Autodesk Fusion 360 part; units mm, degrees
(part 6 of 6)
  line L698 (-62.5, 150.325) -> (-62.5, 137.675)
  arc A698 (-65.675, 134.5) -> (-62.5, 137.675) centre (-65.675, 137.675) ccw
  line L699 (-65.675, 134.5) -> (-78.325, 134.5)
  arc A699 (-81.5, 137.675) -> (-78.325, 134.5) centre (-78.325, 137.675) ccw
  line L700 (-177.5, 137.675) -> (-177.5, 150.325)
  arc A700 (-174.325, 153.5) -> (-177.5, 150.325) centre (-174.325, 150.325) ccw
  line L701 (-174.325, 153.5) -> (-161.675, 153.5)
  arc A701 (-158.5, 150.325) -> (-161.675, 153.5) centre (-161.675, 150.325) ccw
  line L702 (-158.5, 150.325) -> (-158.5, 137.675)
  arc A702 (-161.675, 134.5) -> (-158.5, 137.675) centre (-161.675, 137.675) ccw
  line L703 (-161.675, 134.5) -> (-174.325, 134.5)
  arc A703 (-177.5, 137.675) -> (-174.325, 134.5) centre (-174.325, 137.675) ccw
  line L704 (-105.5, 113.675) -> (-105.5, 126.325)
  arc A704 (-102.325, 129.5) -> (-105.5, 126.325) centre (-102.325, 126.325) ccw
  line L705 (-102.325, 129.5) -> (-89.675, 129.5)
  arc A705 (-86.5, 126.325) -> (-89.675, 129.5) centre (-89.675, 126.325) ccw
  line L706 (-86.5, 126.325) -> (-86.5, 113.675)
  arc A706 (-89.675, 110.5) -> (-86.5, 113.675) centre (-89.675, 113.675) ccw
  line L707 (-89.675, 110.5) -> (-102.325, 110.5)
  arc A707 (-105.5, 113.675) -> (-102.325, 110.5) centre (-102.325, 113.675) ccw
  line L708 (-33.5, 89.675) -> (-33.5, 102.325)
  arc A708 (-30.325, 105.5) -> (-33.5, 102.325) centre (-30.325, 102.325) ccw
  line L709 (-30.325, 105.5) -> (-17.675, 105.5)
  arc A709 (-14.5, 102.325) -> (-17.675, 105.5) centre (-17.675, 102.325) ccw
  line L710 (-14.5, 102.325) -> (-14.5, 89.675)
  arc A710 (-17.675, 86.5) -> (-14.5, 89.675) centre (-17.675, 89.675) ccw
  line L711 (-17.675, 86.5) -> (-30.325, 86.5)
  arc A711 (-33.5, 89.675) -> (-30.325, 86.5) centre (-30.325, 89.675) ccw
  line L712 (-129.5, 89.675) -> (-129.5, 102.325)
  arc A712 (-126.325, 105.5) -> (-129.5, 102.325) centre (-126.325, 102.325) ccw
  line L713 (-126.325, 105.5) -> (-113.675, 105.5)
  arc A713 (-110.5, 102.325) -> (-113.675, 105.5) centre (-113.675, 102.325) ccw
  line L714 (-110.5, 102.325) -> (-110.5, 89.675)
  arc A714 (-113.675, 86.5) -> (-110.5, 89.675) centre (-113.675, 89.675) ccw
  line L715 (-113.675, 86.5) -> (-126.325, 86.5)
  arc A715 (-129.5, 89.675) -> (-126.325, 86.5) centre (-126.325, 89.675) ccw
  line L716 (-57.5, 65.675) -> (-57.5, 78.325)
  arc A716 (-54.325, 81.5) -> (-57.5, 78.325) centre (-54.325, 78.325) ccw
  line L717 (-54.325, 81.5) -> (-41.675, 81.5)
  arc A717 (-38.5, 78.325) -> (-41.675, 81.5) centre (-41.675, 78.325) ccw
  line L718 (-38.5, 78.325) -> (-38.5, 65.675)
  arc A718 (-41.675, 62.5) -> (-38.5, 65.675) centre (-41.675, 65.675) ccw
  line L719 (-41.675, 62.5) -> (-54.325, 62.5)
  arc A719 (-57.5, 65.675) -> (-54.325, 62.5) centre (-54.325, 65.675) ccw
  line L720 (-153.5, 65.675) -> (-153.5, 78.325)
  arc A720 (-150.325, 81.5) -> (-153.5, 78.325) centre (-150.325, 78.325) ccw
  line L721 (-150.325, 81.5) -> (-137.675, 81.5)
  arc A721 (-134.5, 78.325) -> (-137.675, 81.5) centre (-137.675, 78.325) ccw
  line L722 (-134.5, 78.325) -> (-134.5, 65.675)
  arc A722 (-137.675, 62.5) -> (-134.5, 65.675) centre (-137.675, 65.675) ccw
  line L723 (-137.675, 62.5) -> (-150.325, 62.5)
  arc A723 (-153.5, 65.675) -> (-150.325, 62.5) centre (-150.325, 65.675) ccw
  line L724 (-177.5, -54.325) -> (-177.5, -41.675)
  arc A724 (-174.325, -38.5) -> (-177.5, -41.675) centre (-174.325, -41.675) ccw
  line L725 (-174.325, -38.5) -> (-161.675, -38.5)
  arc A725 (-158.5, -41.675) -> (-161.675, -38.5) centre (-161.675, -41.675) ccw
  line L726 (-158.5, -41.675) -> (-158.5, -54.325)
  arc A726 (-161.675, -57.5) -> (-158.5, -54.325) centre (-161.675, -54.325) ccw
  line L727 (-161.675, -57.5) -> (-174.325, -57.5)
  arc A727 (-177.5, -54.325) -> (-174.325, -57.5) centre (-174.325, -54.325) ccw
  line L728 (-129.5, -102.325) -> (-129.5, -89.675)
  arc A728 (-126.325, -86.5) -> (-129.5, -89.675) centre (-126.325, -89.675) ccw
  line L729 (-126.325, -86.5) -> (-113.675, -86.5)
  arc A729 (-110.5, -89.675) -> (-113.675, -86.5) centre (-113.675, -89.675) ccw
  line L730 (-110.5, -89.675) -> (-110.5, -102.325)
  arc A730 (-113.675, -105.5) -> (-110.5, -102.325) centre (-113.675, -102.325) ccw
  line L731 (-113.675, -105.5) -> (-126.325, -105.5)
  arc A731 (-129.5, -102.325) -> (-126.325, -105.5) centre (-126.325, -102.325) ccw
  line L732 (-153.5, -126.325) -> (-153.5, -113.675)
  arc A732 (-150.325, -110.5) -> (-153.5, -113.675) centre (-150.325, -113.675) ccw
  line L733 (-150.325, -110.5) -> (-137.675, -110.5)
  arc A733 (-134.5, -113.675) -> (-137.675, -110.5) centre (-137.675, -113.675) ccw
  line L734 (-134.5, -113.675) -> (-134.5, -126.325)
  arc A734 (-137.675, -129.5) -> (-134.5, -126.325) centre (-137.675, -126.325) ccw
  line L735 (-137.675, -129.5) -> (-150.325, -129.5)
  arc A735 (-153.5, -126.325) -> (-150.325, -129.5) centre (-150.325, -126.325) ccw
  line L736 (-177.5, -150.325) -> (-177.5, -137.675)
  arc A736 (-174.325, -134.5) -> (-177.5, -137.675) centre (-174.325, -137.675) ccw
  line L737 (-174.325, -134.5) -> (-161.675, -134.5)
  arc A737 (-158.5, -137.675) -> (-161.675, -134.5) centre (-161.675, -137.675) ccw
  line L738 (-158.5, -137.675) -> (-158.5, -150.325)
  arc A738 (-161.675, -153.5) -> (-158.5, -150.325) centre (-161.675, -150.325) ccw
  line L739 (-161.675, -153.5) -> (-174.325, -153.5)
  arc A739 (-177.5, -150.325) -> (-174.325, -153.5) centre (-174.325, -150.325) ccw
  line L740 (38.5, -150.325) -> (38.5, -137.675)
  arc A740 (41.675, -134.5) -> (38.5, -137.675) centre (41.675, -137.675) ccw
  line L741 (41.675, -134.5) -> (54.325, -134.5)
  arc A741 (57.5, -137.675) -> (54.325, -134.5) centre (54.325, -137.675) ccw
  line L742 (57.5, -137.675) -> (57.5, -150.325)
  arc A742 (54.325, -153.5) -> (57.5, -150.325) centre (54.325, -150.325) ccw
  line L743 (54.325, -153.5) -> (41.675, -153.5)
  arc A743 (38.5, -150.325) -> (41.675, -153.5) centre (41.675, -150.325) ccw
  line L744 (-81.5, 41.675) -> (-81.5, 54.325)
  arc A744 (-78.325, 57.5) -> (-81.5, 54.325) centre (-78.325, 54.325) ccw
  line L745 (-78.325, 57.5) -> (-65.675, 57.5)
  arc A745 (-62.5, 54.325) -> (-65.675, 57.5) centre (-65.675, 54.325) ccw
  line L746 (-62.5, 54.325) -> (-62.5, 41.675)
  arc A746 (-65.675, 38.5) -> (-62.5, 41.675) centre (-65.675, 41.675) ccw
  line L747 (-65.675, 38.5) -> (-78.325, 38.5)
  arc A747 (-81.5, 41.675) -> (-78.325, 38.5) centre (-78.325, 41.675) ccw
  line L748 (38.5, -174.325) -> (38.5, -161.675)
  arc A748 (41.675, -158.5) -> (38.5, -161.675) centre (41.675, -161.675) ccw
  line L749 (41.675, -158.5) -> (54.325, -158.5)
  arc A749 (57.5, -161.675) -> (54.325, -158.5) centre (54.325, -161.675) ccw
  line L750 (57.5, -161.675) -> (57.5, -174.325)
  arc A750 (54.325, -177.5) -> (57.5, -174.325) centre (54.325, -174.325) ccw
  line L751 (54.325, -177.5) -> (41.675, -177.5)
  arc A751 (38.5, -174.325) -> (41.675, -177.5) centre (41.675, -174.325) ccw
  line L752 (-105.5, -150.325) -> (-105.5, -137.675)
  arc A752 (-102.325, -134.5) -> (-105.5, -137.675) centre (-102.325, -137.675) ccw
  line L753 (-102.325, -134.5) -> (-89.675, -134.5)
  arc A753 (-86.5, -137.675) -> (-89.675, -134.5) centre (-89.675, -137.675) ccw
  line L754 (-86.5, -137.675) -> (-86.5, -150.325)
  arc A754 (-89.675, -153.5) -> (-86.5, -150.325) centre (-89.675, -150.325) ccw
  line L755 (-89.675, -153.5) -> (-102.325, -153.5)
  arc A755 (-105.5, -150.325) -> (-102.325, -153.5) centre (-102.325, -150.325) ccw
  line L756 (-57.5, 41.675) -> (-57.5, 54.325)
  arc A756 (-54.325, 57.5) -> (-57.5, 54.325) centre (-54.325, 54.325) ccw
  line L757 (-54.325, 57.5) -> (-41.675, 57.5)
  arc A757 (-38.5, 54.325) -> (-41.675, 57.5) centre (-41.675, 54.325) ccw
  line L758 (-38.5, 54.325) -> (-38.5, 41.675)
  arc A758 (-41.675, 38.5) -> (-38.5, 41.675) centre (-41.675, 41.675) ccw
  line L759 (-41.675, 38.5) -> (-54.325, 38.5)
  arc A759 (-57.5, 41.675) -> (-54.325, 38.5) centre (-54.325, 41.675) ccw
  line L760 (-129.5, -30.325) -> (-129.5, -17.675)
  arc A760 (-126.325, -14.5) -> (-129.5, -17.675) centre (-126.325, -17.675) ccw
  line L761 (-126.325, -14.5) -> (-113.675, -14.5)
  arc A761 (-110.5, -17.675) -> (-113.675, -14.5) centre (-113.675, -17.675) ccw
  line L762 (-110.5, -17.675) -> (-110.5, -30.325)
  arc A762 (-113.675, -33.5) -> (-110.5, -30.325) centre (-113.675, -30.325) ccw
  line L763 (-113.675, -33.5) -> (-126.325, -33.5)
  arc A763 (-129.5, -30.325) -> (-126.325, -33.5) centre (-126.325, -30.325) ccw
  line L764 (-105.5, -102.325) -> (-105.5, -89.675)
  arc A764 (-102.325, -86.5) -> (-105.5, -89.675) centre (-102.325, -89.675) ccw
  line L765 (-102.325, -86.5) -> (-89.675, -86.5)
  arc A765 (-86.5, -89.675) -> (-89.675, -86.5) centre (-89.675, -89.675) ccw
  line L766 (-86.5, -89.675) -> (-86.5, -102.325)
  arc A766 (-89.675, -105.5) -> (-86.5, -102.325) centre (-89.675, -102.325) ccw
  line L767 (-89.675, -105.5) -> (-102.325, -105.5)
  arc A767 (-105.5, -102.325) -> (-102.325, -105.5) centre (-102.325, -102.325) ccw
  line L768 (62.5, 161.675) -> (62.5, 174.325)
  arc A768 (65.675, 177.5) -> (62.5, 174.325) centre (65.675, 174.325) ccw
  line L769 (65.675, 177.5) -> (78.325, 177.5)
  arc A769 (81.5, 174.325) -> (78.325, 177.5) centre (78.325, 174.325) ccw
  line L770 (81.5, 174.325) -> (81.5, 161.675)
  arc A770 (78.325, 158.5) -> (81.5, 161.675) centre (78.325, 161.675) ccw
  line L771 (78.325, 158.5) -> (65.675, 158.5)
  arc A771 (62.5, 161.675) -> (65.675, 158.5) centre (65.675, 161.675) ccw
  line L772 (62.5, 137.675) -> (62.5, 150.325)
  arc A772 (65.675, 153.5) -> (62.5, 150.325) centre (65.675, 150.325) ccw
  line L773 (65.675, 153.5) -> (78.325, 153.5)
  arc A773 (81.5, 150.325) -> (78.325, 153.5) centre (78.325, 150.325) ccw
  line L774 (81.5, 150.325) -> (81.5, 137.675)
  arc A774 (78.325, 134.5) -> (81.5, 137.675) centre (78.325, 137.675) ccw
  line L775 (78.325, 134.5) -> (65.675, 134.5)
  arc A775 (62.5, 137.675) -> (65.675, 134.5) centre (65.675, 137.675) ccw
  line L776 (62.5, 113.675) -> (62.5, 126.325)
  arc A776 (65.675, 129.5) -> (62.5, 126.325) centre (65.675, 126.325) ccw
  line L777 (65.675, 129.5) -> (78.325, 129.5)
  arc A777 (81.5, 126.325) -> (78.325, 129.5) centre (78.325, 126.325) ccw
  line L778 (81.5, 126.325) -> (81.5, 113.675)
  arc A778 (78.325, 110.5) -> (81.5, 113.675) centre (78.325, 113.675) ccw
  line L779 (78.325, 110.5) -> (65.675, 110.5)
  arc A779 (62.5, 113.675) -> (65.675, 110.5) centre (65.675, 113.675) ccw
  line L780 (62.5, 89.675) -> (62.5, 102.325)
  arc A780 (65.675, 105.5) -> (62.5, 102.325) centre (65.675, 102.325) ccw
  line L781 (65.675, 105.5) -> (78.325, 105.5)
  arc A781 (81.5, 102.325) -> (78.325, 105.5) centre (78.325, 102.325) ccw
  line L782 (81.5, 102.325) -> (81.5, 89.675)
  arc A782 (78.325, 86.5) -> (81.5, 89.675) centre (78.325, 89.675) ccw
  line L783 (78.325, 86.5) -> (65.675, 86.5)
  arc A783 (62.5, 89.675) -> (65.675, 86.5) centre (65.675, 89.675) ccw
  line L784 (62.5, 65.675) -> (62.5, 78.325)
  arc A784 (65.675, 81.5) -> (62.5, 78.325) centre (65.675, 78.325) ccw
  line L785 (65.675, 81.5) -> (78.325, 81.5)
  arc A785 (81.5, 78.325) -> (78.325, 81.5) centre (78.325, 78.325) ccw
  line L786 (81.5, 78.325) -> (81.5, 65.675)
  arc A786 (78.325, 62.5) -> (81.5, 65.675) centre (78.325, 65.675) ccw
  line L787 (78.325, 62.5) -> (65.675, 62.5)
  arc A787 (62.5, 65.675) -> (65.675, 62.5) centre (65.675, 65.675) ccw
  line L788 (-9.5, 65.675) -> (-9.5, 78.325)
  arc A788 (-6.325, 81.5) -> (-9.5, 78.325) centre (-6.325, 78.325) ccw
  line L789 (-6.325, 81.5) -> (6.325, 81.5)
  arc A789 (9.5, 78.325) -> (6.325, 81.5) centre (6.325, 78.325) ccw
  line L790 (9.5, 78.325) -> (9.5, 65.675)
  arc A790 (6.325, 62.5) -> (9.5, 65.675) centre (6.325, 65.675) ccw
  line L791 (6.325, 62.5) -> (-6.325, 62.5)
  arc A791 (-9.5, 65.675) -> (-6.325, 62.5) centre (-6.325, 65.675) ccw
  line L792 (-9.5, 41.675) -> (-9.5, 54.325)
  arc A792 (-6.325, 57.5) -> (-9.5, 54.325) centre (-6.325, 54.325) ccw
  line L793 (-6.325, 57.5) -> (6.325, 57.5)
  arc A793 (9.5, 54.325) -> (6.325, 57.5) centre (6.325, 54.325) ccw
  line L794 (9.5, 54.325) -> (9.5, 41.675)
  arc A794 (6.325, 38.5) -> (9.5, 41.675) centre (6.325, 41.675) ccw
  line L795 (6.325, 38.5) -> (-6.325, 38.5)
  arc A795 (-9.5, 41.675) -> (-6.325, 38.5) centre (-6.325, 41.675) ccw
  line L796 (-9.5, 17.675) -> (-9.5, 30.325)
  arc A796 (-6.325, 33.5) -> (-9.5, 30.325) centre (-6.325, 30.325) ccw
  line L797 (-6.325, 33.5) -> (6.325, 33.5)
  arc A797 (9.5, 30.325) -> (6.325, 33.5) centre (6.325, 30.325) ccw
  line L798 (9.5, 30.325) -> (9.5, 17.675)
  arc A798 (6.325, 14.5) -> (9.5, 17.675) centre (6.325, 17.675) ccw
  line L799 (6.325, 14.5) -> (-6.325, 14.5)
  arc A799 (-9.5, 17.675) -> (-6.325, 14.5) centre (-6.325, 17.675) ccw
  line L800 (9.5, 6.325) -> (9.5, -6.325)
  arc A800 (6.325, -9.5) -> (9.5, -6.325) centre (6.325, -6.325) ccw
  line L801 (6.325, -9.5) -> (-6.325, -9.5)
  arc A801 (-9.5, -6.325) -> (-6.325, -9.5) centre (-6.325, -6.325) ccw
  line L802 (-9.5, -6.325) -> (-9.5, 6.325)
  arc A802 (-6.325, 9.5) -> (-9.5, 6.325) centre (-6.325, 6.325) ccw
  line L803 (-6.325, 9.5) -> (6.325, 9.5)
  arc A803 (9.5, 6.325) -> (6.325, 9.5) centre (6.325, 6.325) ccw
  line L804 (158.5, 137.675) -> (158.5, 150.325)
  arc A804 (161.675, 153.5) -> (158.5, 150.325) centre (161.675, 150.325) ccw
  line L805 (161.675, 153.5) -> (174.325, 153.5)
  arc A805 (177.5, 150.325) -> (174.325, 153.5) centre (174.325, 150.325) ccw
  line L806 (177.5, 150.325) -> (177.5, 137.675)
  arc A806 (174.325, 134.5) -> (177.5, 137.675) centre (174.325, 137.675) ccw
  line L807 (174.325, 134.5) -> (161.675, 134.5)
  arc A807 (158.5, 137.675) -> (161.675, 134.5) centre (161.675, 137.675) ccw
  line L808 (158.5, 113.675) -> (158.5, 126.325)
  arc A808 (161.675, 129.5) -> (158.5, 126.325) centre (161.675, 126.325) ccw
  line L809 (161.675, 129.5) -> (174.325, 129.5)
  arc A809 (177.5, 126.325) -> (174.325, 129.5) centre (174.325, 126.325) ccw
  line L810 (177.5, 126.325) -> (177.5, 113.675)
  arc A810 (174.325, 110.5) -> (177.5, 113.675) centre (174.325, 113.675) ccw
  line L811 (174.325, 110.5) -> (161.675, 110.5)
  arc A811 (158.5, 113.675) -> (161.675, 110.5) centre (161.675, 113.675) ccw
  line L812 (158.5, 89.675) -> (158.5, 102.325)
  arc A812 (161.675, 105.5) -> (158.5, 102.325) centre (161.675, 102.325) ccw
  line L813 (161.675, 105.5) -> (174.325, 105.5)
  arc A813 (177.5, 102.325) -> (174.325, 105.5) centre (174.325, 102.325) ccw
  line L814 (177.5, 102.325) -> (177.5, 89.675)
  arc A814 (174.325, 86.5) -> (177.5, 89.675) centre (174.325, 89.675) ccw
  line L815 (174.325, 86.5) -> (161.675, 86.5)
  arc A815 (158.5, 89.675) -> (161.675, 86.5) centre (161.675, 89.675) ccw
  line L816 (158.5, 65.675) -> (158.5, 78.325)
  arc A816 (161.675, 81.5) -> (158.5, 78.325) centre (161.675, 78.325) ccw
  line L817 (161.675, 81.5) -> (174.325, 81.5)
  arc A817 (177.5, 78.325) -> (174.325, 81.5) centre (174.325, 78.325) ccw
  line L818 (177.5, 78.325) -> (177.5, 65.675)
  arc A818 (174.325, 62.5) -> (177.5, 65.675) centre (174.325, 65.675) ccw
  line L819 (174.325, 62.5) -> (161.675, 62.5)
  arc A819 (158.5, 65.675) -> (161.675, 62.5) centre (161.675, 65.675) ccw
  line L820 (158.5, 41.675) -> (158.5, 54.325)
  arc A820 (161.675, 57.5) -> (158.5, 54.325) centre (161.675, 54.325) ccw
  line L821 (161.675, 57.5) -> (174.325, 57.5)
  arc A821 (177.5, 54.325) -> (174.325, 57.5) centre (174.325, 54.325) ccw
  line L822 (177.5, 54.325) -> (177.5, 41.675)
  arc A822 (174.325, 38.5) -> (177.5, 41.675) centre (174.325, 41.675) ccw
  line L823 (174.325, 38.5) -> (161.675, 38.5)
  arc A823 (158.5, 41.675) -> (161.675, 38.5) centre (161.675, 41.675) ccw
  line L824 (158.5, 17.675) -> (158.5, 30.325)
  arc A824 (161.675, 33.5) -> (158.5, 30.325) centre (161.675, 30.325) ccw
  line L825 (161.675, 33.5) -> (174.325, 33.5)
  arc A825 (177.5, 30.325) -> (174.325, 33.5) centre (174.325, 30.325) ccw
  line L826 (177.5, 30.325) -> (177.5, 17.675)
  arc A826 (174.325, 14.5) -> (177.5, 17.675) centre (174.325, 17.675) ccw
  line L827 (174.325, 14.5) -> (161.675, 14.5)
  arc A827 (158.5, 17.675) -> (161.675, 14.5) centre (161.675, 17.675) ccw
  line L828 (158.5, -6.325) -> (158.5, 6.325)
  arc A828 (161.675, 9.5) -> (158.5, 6.325) centre (161.675, 6.325) ccw
  line L829 (161.675, 9.5) -> (174.325, 9.5)
  arc A829 (177.5, 6.325) -> (174.325, 9.5) centre (174.325, 6.325) ccw
  line L830 (177.5, 6.325) -> (177.5, -6.325)
  arc A830 (174.325, -9.5) -> (177.5, -6.325) centre (174.325, -6.325) ccw
  line L831 (174.325, -9.5) -> (161.675, -9.5)
  arc A831 (158.5, -6.325) -> (161.675, -9.5) centre (161.675, -6.325) ccw
  line L832 (62.5, -30.325) -> (62.5, -17.675)
  arc A832 (65.675, -14.5) -> (62.5, -17.675) centre (65.675, -17.675) ccw
  line L833 (65.675, -14.5) -> (78.325, -14.5)
  arc A833 (81.5, -17.675) -> (78.325, -14.5) centre (78.325, -17.675) ccw
  line L834 (81.5, -17.675) -> (81.5, -30.325)
  arc A834 (78.325, -33.5) -> (81.5, -30.325) centre (78.325, -30.325) ccw
  line L835 (78.325, -33.5) -> (65.675, -33.5)
  arc A835 (62.5, -30.325) -> (65.675, -33.5) centre (65.675, -30.325) ccw
  line L836 (62.5, -54.325) -> (62.5, -41.675)
  arc A836 (65.675, -38.5) -> (62.5, -41.675) centre (65.675, -41.675) ccw
  line L837 (65.675, -38.5) -> (78.325, -38.5)
  arc A837 (81.5, -41.675) -> (78.325, -38.5) centre (78.325, -41.675) ccw
  line L838 (81.5, -41.675) -> (81.5, -54.325)
  arc A838 (78.325, -57.5) -> (81.5, -54.325) centre (78.325, -54.325) ccw
  line L839 (78.325, -57.5) -> (65.675, -57.5)
  arc A839 (62.5, -54.325) -> (65.675, -57.5) centre (65.675, -54.325) ccw
  line L840 (14.5, -102.325) -> (14.5, -89.675)
  arc A840 (17.675, -86.5) -> (14.5, -89.675) centre (17.675, -89.675) ccw
  line L841 (17.675, -86.5) -> (30.325, -86.5)
  arc A841 (33.5, -89.675) -> (30.325, -86.5) centre (30.325, -89.675) ccw
  line L842 (33.5, -89.675) -> (33.5, -102.325)
  arc A842 (30.325, -105.5) -> (33.5, -102.325) centre (30.325, -102.325) ccw
  line L843 (30.325, -105.5) -> (17.675, -105.5)
  arc A843 (14.5, -102.325) -> (17.675, -105.5) centre (17.675, -102.325) ccw
  line L844 (158.5, -78.325) -> (158.5, -65.675)
  arc A844 (161.675, -62.5) -> (158.5, -65.675) centre (161.675, -65.675) ccw
  line L845 (161.675, -62.5) -> (174.325, -62.5)
  arc A845 (177.5, -65.675) -> (174.325, -62.5) centre (174.325, -65.675) ccw
  line L846 (177.5, -65.675) -> (177.5, -78.325)
  arc A846 (174.325, -81.5) -> (177.5, -78.325) centre (174.325, -78.325) ccw
  line L847 (174.325, -81.5) -> (161.675, -81.5)
  arc A847 (158.5, -78.325) -> (161.675, -81.5) centre (161.675, -78.325) ccw
  line L848 (-81.5, 17.675) -> (-81.5, 30.325)
  arc A848 (-78.325, 33.5) -> (-81.5, 30.325) centre (-78.325, 30.325) ccw
  line L849 (-78.325, 33.5) -> (-65.675, 33.5)
  arc A849 (-62.5, 30.325) -> (-65.675, 33.5) centre (-65.675, 30.325) ccw
  line L850 (-62.5, 30.325) -> (-62.5, 17.675)
  arc A850 (-65.675, 14.5) -> (-62.5, 17.675) centre (-65.675, 17.675) ccw
  line L851 (-65.675, 14.5) -> (-78.325, 14.5)
  arc A851 (-81.5, 17.675) -> (-78.325, 14.5) centre (-78.325, 17.675) ccw
  line L852 (14.5, -78.325) -> (14.5, -65.675)
  arc A852 (17.675, -62.5) -> (14.5, -65.675) centre (17.675, -65.675) ccw
  line L853 (17.675, -62.5) -> (30.325, -62.5)
  arc A853 (33.5, -65.675) -> (30.325, -62.5) centre (30.325, -65.675) ccw
  line L854 (33.5, -65.675) -> (33.5, -78.325)
  arc A854 (30.325, -81.5) -> (33.5, -78.325) centre (30.325, -78.325) ccw
  line L855 (30.325, -81.5) -> (17.675, -81.5)
  arc A855 (14.5, -78.325) -> (17.675, -81.5) centre (17.675, -78.325) ccw
  line L856 (-177.5, -6.325) -> (-177.5, 6.325)
  arc A856 (-174.325, 9.5) -> (-177.5, 6.325) centre (-174.325, 6.325) ccw
  line L857 (-174.325, 9.5) -> (-161.675, 9.5)
  arc A857 (-158.5, 6.325) -> (-161.675, 9.5) centre (-161.675, 6.325) ccw
  line L858 (-158.5, 6.325) -> (-158.5, -6.325)
  arc A858 (-161.675, -9.5) -> (-158.5, -6.325) centre (-161.675, -6.325) ccw
  line L859 (-161.675, -9.5) -> (-174.325, -9.5)
  arc A859 (-177.5, -6.325) -> (-174.325, -9.5) centre (-174.325, -6.325) ccw
  line L860 (-153.5, -6.325) -> (-153.5, 6.325)
  arc A860 (-150.325, 9.5) -> (-153.5, 6.325) centre (-150.325, 6.325) ccw
  line L861 (-150.325, 9.5) -> (-137.675, 9.5)
  arc A861 (-134.5, 6.325) -> (-137.675, 9.5) centre (-137.675, 6.325) ccw
  line L862 (-134.5, 6.325) -> (-134.5, -6.325)
  arc A862 (-137.675, -9.5) -> (-134.5, -6.325) centre (-137.675, -6.325) ccw
  line L863 (-137.675, -9.5) -> (-150.325, -9.5)
  arc A863 (-153.5, -6.325) -> (-150.325, -9.5) centre (-150.325, -6.325) ccw
  line L864 (-105.5, -6.325) -> (-105.5, 6.325)
  arc A864 (-102.325, 9.5) -> (-105.5, 6.325) centre (-102.325, 6.325) ccw
  line L865 (-102.325, 9.5) -> (-89.675, 9.5)
  arc A865 (-86.5, 6.325) -> (-89.675, 9.5) centre (-89.675, 6.325) ccw
  line L866 (-86.5, 6.325) -> (-86.5, -6.325)
  arc A866 (-89.675, -9.5) -> (-86.5, -6.325) centre (-89.675, -6.325) ccw
  line L867 (-89.675, -9.5) -> (-102.325, -9.5)
  arc A867 (-105.5, -6.325) -> (-102.325, -9.5) centre (-102.325, -6.325) ccw
  line L868 (134.5, -54.325) -> (134.5, -41.675)
  arc A868 (137.675, -38.5) -> (134.5, -41.675) centre (137.675, -41.675) ccw
  line L869 (137.675, -38.5) -> (150.325, -38.5)
  arc A869 (153.5, -41.675) -> (150.325, -38.5) centre (150.325, -41.675) ccw
  line L870 (153.5, -41.675) -> (153.5, -54.325)
  arc A870 (150.325, -57.5) -> (153.5, -54.325) centre (150.325, -54.325) ccw
  line L871 (150.325, -57.5) -> (137.675, -57.5)
  arc A871 (134.5, -54.325) -> (137.675, -57.5) centre (137.675, -54.325) ccw
  line L872 (86.5, -30.325) -> (86.5, -17.675)
  arc A872 (89.675, -14.5) -> (86.5, -17.675) centre (89.675, -17.675) ccw
  line L873 (89.675, -14.5) -> (102.325, -14.5)
  arc A873 (105.5, -17.675) -> (102.325, -14.5) centre (102.325, -17.675) ccw
  line L874 (105.5, -17.675) -> (105.5, -30.325)
  arc A874 (102.325, -33.5) -> (105.5, -30.325) centre (102.325, -30.325) ccw
  line L875 (102.325, -33.5) -> (89.675, -33.5)
  arc A875 (86.5, -30.325) -> (89.675, -33.5) centre (89.675, -30.325) ccw
  line L876 (158.5, -30.325) -> (158.5, -17.675)
  arc A876 (161.675, -14.5) -> (158.5, -17.675) centre (161.675, -17.675) ccw
  line L877 (161.675, -14.5) -> (174.325, -14.5)
  arc A877 (177.5, -17.675) -> (174.325, -14.5) centre (174.325, -17.675) ccw
  line L878 (177.5, -17.675) -> (177.5, -30.325)
  arc A878 (174.325, -33.5) -> (177.5, -30.325) centre (174.325, -30.325) ccw
  line L879 (174.325, -33.5) -> (161.675, -33.5)
  arc A879 (158.5, -30.325) -> (161.675, -33.5) centre (161.675, -30.325) ccw
  line L880 (-57.5, -126.325) -> (-57.5, -113.675)
  arc A880 (-54.325, -110.5) -> (-57.5, -113.675) centre (-54.325, -113.675) ccw
  line L881 (-54.325, -110.5) -> (-41.675, -110.5)
  arc A881 (-38.5, -113.675) -> (-41.675, -110.5) centre (-41.675, -113.675) ccw
  line L882 (-38.5, -113.675) -> (-38.5, -126.325)
  arc A882 (-41.675, -129.5) -> (-38.5, -126.325) centre (-41.675, -126.325) ccw
  line L883 (-41.675, -129.5) -> (-54.325, -129.5)
  arc A883 (-57.5, -126.325) -> (-54.325, -129.5) centre (-54.325, -126.325) ccw
  line L884 (-81.5, -174.325) -> (-81.5, -161.675)
  arc A884 (-78.325, -158.5) -> (-81.5, -161.675) centre (-78.325, -161.675) ccw
  line L885 (-78.325, -158.5) -> (-65.675, -158.5)
  arc A885 (-62.5, -161.675) -> (-65.675, -158.5) centre (-65.675, -161.675) ccw
  line L886 (-62.5, -161.675) -> (-62.5, -174.325)
  arc A886 (-65.675, -177.5) -> (-62.5, -174.325) centre (-65.675, -174.325) ccw
  line L887 (-65.675, -177.5) -> (-78.325, -177.5)
  arc A887 (-81.5, -174.325) -> (-78.325, -177.5) centre (-78.325, -174.325) ccw
  line L888 (-57.5, -78.325) -> (-57.5, -65.675)
  arc A888 (-54.325, -62.5) -> (-57.5, -65.675) centre (-54.325, -65.675) ccw
  line L889 (-54.325, -62.5) -> (-41.675, -62.5)
  arc A889 (-38.5, -65.675) -> (-41.675, -62.5) centre (-41.675, -65.675) ccw
  line L890 (-38.5, -65.675) -> (-38.5, -78.325)
  arc A890 (-41.675, -81.5) -> (-38.5, -78.325) centre (-41.675, -78.325) ccw
  line L891 (-41.675, -81.5) -> (-54.325, -81.5)
  arc A891 (-57.5, -78.325) -> (-54.325, -81.5) centre (-54.325, -78.325) ccw
  line L892 (-105.5, -54.325) -> (-105.5, -41.675)
  arc A892 (-102.325, -38.5) -> (-105.5, -41.675) centre (-102.325, -41.675) ccw
  line L893 (-102.325, -38.5) -> (-89.675, -38.5)
  arc A893 (-86.5, -41.675) -> (-89.675, -38.5) centre (-89.675, -41.675) ccw
  line L894 (-86.5, -41.675) -> (-86.5, -54.325)
  arc A894 (-89.675, -57.5) -> (-86.5, -54.325) centre (-89.675, -54.325) ccw
  line L895 (-89.675, -57.5) -> (-102.325, -57.5)
  arc A895 (-105.5, -54.325) -> (-102.325, -57.5) centre (-102.325, -54.325) ccw
  line L896 (38.5, -78.325) -> (38.5, -65.675)
  arc A896 (41.675, -62.5) -> (38.5, -65.675) centre (41.675, -65.675) ccw
  line L897 (41.675, -62.5) -> (54.325, -62.5)
  arc A897 (57.5, -65.675) -> (54.325, -62.5) centre (54.325, -65.675) ccw
  line L898 (57.5, -65.675) -> (57.5, -78.325)
  arc A898 (54.325, -81.5) -> (57.5, -78.325) centre (54.325, -78.325) ccw
  line L899 (54.325, -81.5) -> (41.675, -81.5)
  arc A899 (38.5, -78.325) -> (41.675, -81.5) centre (41.675, -78.325) ccw
  line L900 (-234, 234) -> (-234, -234)
  line L901 (-234, -234) -> (234, -234)
  line L902 (234, -234) -> (234, 234)
  line L903 (234, 234) -> (-234, 234)
  line L904 (263.4694, -51.681) -> (325, -51.681)
  line L905 (325, -51.681) -> (325, 75)
  line L906 (325, 75) -> (263.4694, 75)
  line L907 (263.4694, 75) -> (263.4694, -51.681)
  line L908 (185.0931, 107.3955) -> (107.6544, 107.3955)
  line L909 (107.6544, 107.3955) -> (107.6544, 184.5967)
  line L910 (107.6544, 184.5967) -> (185.0931, 184.5967)
  line L911 (185.0931, 184.5967) -> (185.0931, 107.3955)
  dimension "d51" = 61.5306
  dimension "d52" = 77.4387
  constraint horizontal L904
  constraint vertical L905
  constraint horizontal L906
  constraint vertical L907
  constraint horizontal L908
  constraint vertical L909
  constraint horizontal L910
  constraint vertical L911
sketch "Sketch3" plane through (0, 0, 0) normal (1, 0, 0) x (0, 0, -1)
sketch "Sketch4" plane through (0, 0, 0) normal (0, -1, 0) x (1, 0, 0)
  line L0 (-254, -254) -> (254, -254)
  line L1 (254, -254) -> (254, 254)
  line L2 (254, 254) -> (-254, 254)
  line L3 (-254, 254) -> (-254, -254)
  line L4 (7.6921, 250.9646) -> (-5.0079, 250.9646)
  line L5 (-5.0079, 250.9646) -> (-5.0079, 276.3646)
  line L6 (-5.0079, 276.3646) -> (7.6921, 276.3646)
  line L7 (7.6921, 276.3646) -> (7.6921, 250.9646)
  line L8 (7.6921, 250.9646) -> (-5.0079, 276.3646) construction
  line L9 (-5.0079, 250.9646) -> (7.6921, 276.3646) construction
  line L10 (-277.3529, -6.3611) -> (-251.9529, -6.3611)
  line L11 (-251.9529, -6.3611) -> (-251.9529, 6.3389)
  line L12 (-251.9529, 6.3389) -> (-277.3529, 6.3389)
  line L13 (-277.3529, 6.3389) -> (-277.3529, -6.3611)
  line L14 (-277.3529, -6.3611) -> (-251.9529, 6.3389) construction
  line L15 (-251.9529, -6.3611) -> (-277.3529, 6.3389) construction
  line L16 (250.8821, 6.35) -> (276.2821, 6.35)
  line L17 (276.2821, 6.35) -> (276.2821, -6.35)
  line L18 (276.2821, -6.35) -> (250.8821, -6.35)
  line L19 (250.8821, -6.35) -> (250.8821, 6.35)
  line L20 (250.8821, 6.35) -> (276.2821, -6.35) construction
  line L21 (276.2821, 6.35) -> (250.8821, -6.35) construction
  line L22 (-6.0932, -275.6546) -> (6.6068, -275.6546)
  line L23 (6.6068, -275.6546) -> (6.6068, -250.2546)
  line L24 (6.6068, -250.2546) -> (-6.0932, -250.2546)
  line L25 (-6.0932, -250.2546) -> (-6.0932, -275.6546)
  line L26 (-6.0932, -275.6546) -> (6.6068, -250.2546) construction
  line L27 (6.6068, -275.6546) -> (-6.0932, -250.2546) construction
  point P0 (83089.3058, 0)
  dimension "d33" = 25.4
  dimension "d34" = 12.7
  dimension "d35" = 25.4
  dimension "d36" = 12.7
  dimension "d39" = 25.4
  dimension "d40" = 12.7
  dimension "d41" = 25.4
  dimension "d42" = 12.7
  constraint perpendicular L4 L5
  constraint parallel L4 L6
  constraint parallel L5 L7
  constraint horizontal L4
  constraint coincident L8
  constraint coincident L9
  constraint midpoint L9
  constraint perpendicular L10 L11
  constraint parallel L10 L12
  constraint parallel L11 L13
  constraint horizontal L10
  constraint coincident L14 P0
  constraint coincident L15 P0
  constraint midpoint L15 P0
  constraint perpendicular L16 L17
  constraint parallel L16 L18
  constraint parallel L17 L19
  constraint horizontal L16
  constraint coincident L20 origin
  constraint coincident L21 origin
  constraint midpoint L20 origin
  constraint perpendicular L22 L23
  constraint parallel L22 L24
  constraint parallel L23 L25
  constraint horizontal L22
  constraint coincident L26 origin
  constraint coincident L27 origin
  measures "d41" distance of origin
extrude "Extrude9" [suppressed]
extrude "Extrude10" [suppressed]
extrude "Extrude11" [suppressed]
extrude "Extrude12" [suppressed]
equation "extra_depth = 3 mm"
equation "d19 = -extra_depth"
equation "d21 = -extra_depth"
equation "d23 = -extra_depth"
equation "d25 = -extra_depth"
equation "d27 = -extra_depth"
